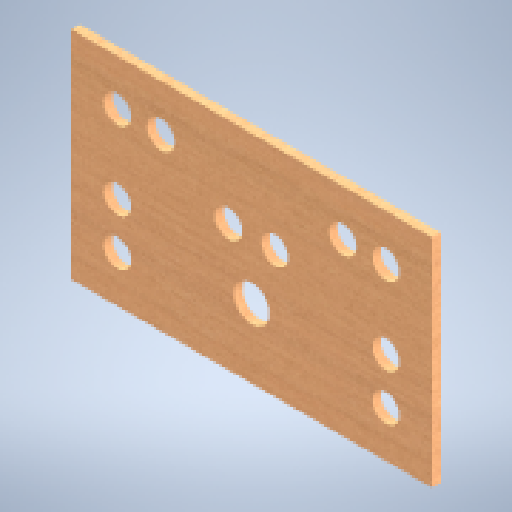
# Autodesk Inventor part: Grundplatte_Konsole
Saved by Autodesk Inventor 2024 (Build 280153000, 153)
## iProperties
Created: 2024-05-02
Part Number: Grundplatte_Konsole
Material: Holz (Kirsche)
Document SubType Name: Modeling
Designer: haniv
Density: 0.63 g/cm^3
Appearance: Kirsche - natur - schwacher Glanz
Author: haniv
Autodesk Inventor part; units mm, degrees
ref_plane "YZ Plane" through (0, 0, 0) normal (1, 0, 0) x (0, 1, 0)
ref_plane "XZ Plane" through (0, 0, 0) normal (0, 1, 0) x (-1, 0, 0)
ref_plane "XY Plane" through (0, 0, 0) normal (0, 0, 1) x (1, 0, 0)
sketch "Skizze1" plane through (0, 0, 0) normal (0, 1, 0) x (-1, 0, 0)
  line L0 (125, 75) -> (-125, 75)
  line L1 (-125, 75) -> (-125, -75)
  line L2 (-125, -75) -> (125, -75)
  line L3 (125, -75) -> (125, 75)
  point P0 (0, 0)
  point P1 (0, -75)
  point P2 (125, 0)
  dimension "d0" = 250
  dimension "d1" = 150
  constraints: 8 end point, 2 midpoint, 2 parallel, 1 horizontal, 1 horizontal alignment, 1 perpendicular, 1 vertical alignment
  measures "d0" distance of L2.end L1.end
  measures "d1" distance of L1.end L0.end
extrude "Extrusion1" add sketch "Skizze1" along normal blind 6
sketch "Skizze2" plane through (0, 0, 0) normal (0, -1, 0) x (1, 0, 0)
  circle A0 centre (0, -38) radius 12.5
  circle A1 centre (-93, -43) radius 9.5
  circle A2 centre (-93, -11) radius 9.5
  circle A3 centre (93, -43) radius 9.5
  circle A4 centre (93, -11) radius 9.5
  circle A5 centre (93, 43) radius 9.5
  circle A6 centre (-63, 43) radius 9.5
  circle A7 centre (63, 43) radius 9.5
  circle A8 centre (-93, 43) radius 9.5
  line L0 (125, 75) -> (125, -75) projected
  line L1 (-125, 75) -> (125, 75) projected
  line L2 (-125, -75) -> (-125, 75) projected
  line L3 (125, -75) -> (-125, -75) projected
  line L4 (-113, 63) -> (113, 63) construction
  line L5 (113, 63) -> (113, -63) construction
  line L6 (113, -63) -> (-113, -63) construction
  line L7 (-113, -63) -> (-113, 63) construction
  line L8 (-93, -11) -> (-93, -43) construction
  line L9 (93, -11) -> (93, -43) construction
  circle A9 centre (93, -43) radius 12.5 construction
  circle A10 centre (93, 43) radius 12.5 construction
  circle A11 centre (63, 43) radius 12.5 construction
  circle A12 centre (0, 43) radius 9.5
  circle A13 centre (0, 11) radius 9.5
  line L10 (0, 43) -> (0, 11) construction
  circle A14 centre (0, -38) radius 16 construction
  point P0 (0, 0)
  point P1 (93, -27)
  point P2 (-93, -27)
  point P3 (0, 10.7432)
  point P4 (0, -63)
  dimension "d4" = 25
  dimension "d5" = 19
  dimension "d6" = 19
  dimension "d7" = 19
  dimension "d8" = 19
  dimension "d9" = 19
  dimension "d10" = 19
  dimension "d11" = 19
  dimension "d12" = 19
  dimension "d13" = 12
  dimension "d14" = 12
  dimension "d15" = 12
  dimension "d16" = 12
  dimension "d19" = 32
  dimension "d20" = 20
  dimension "d21" = 20
  dimension "d22" = 20
  dimension "d23" = 25
  dimension "d25" = 20
  dimension "d26" = 25
  dimension "d27" = 25
  dimension "d28" = 30
  dimension "d30" = 30
  dimension "d33" = 32
  dimension "d34" = 25
  constraints: 15 centre point, 14 end point, 7 vertical alignment, 5 horizontal alignment, 4 coincident, 4 parallel, 3 midpoint, 3 vertical, 2 equal radius, 1 horizontal, 1 perpendicular
  measures "d4" diameter of A0
  measures "d5" diameter of A1
  measures "d6" diameter of A2
  measures "d7" diameter of A3
  measures "d8" diameter of A4
  measures "d9" diameter of A5
  measures "d10" diameter of A6
  measures "d11" diameter of A7
  measures "d12" diameter of A8
  measures "d13" distance between parallel lines of L1 L4
  measures "d14" distance between parallel lines of L2 L7
  measures "d15" distance between parallel lines of L3 L6
  measures "d16" distance between parallel lines of L0 L5
  measures "d19" distance of L9.start L9.end
  measures "d20" distance from line of L6 L9.end
  measures "d21" distance from line of L5 L9.end
  measures "d22" distance between parallel lines of L7 L8
  measures "d23" diameter of A9
  measures "d25" distance from line of L4 A5.centre
  measures "d26" diameter of A10
  measures "d27" diameter of A11
  measures "d28" distance of A5.centre A7.centre
  measures "d30" distance of A8.centre A6.centre
  measures "d33" diameter of A14
  measures "d34" distance of point (0, -63) A14.centre
extrude "Extrusion2" cut sketch "Skizze2" against normal through all contours A0 | A1 | A2 | A3 | A4 | A5 | A6 | A7 | A8 | A12 | A13
